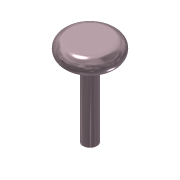
# Autodesk Inventor part: screw
Saved by Autodesk Inventor 2022 Beta2 (Build 260130000, 130) ContinuousBuild 0
## iProperties
Shininess: 64.0
Length Units: 11272
Angle Units: 11279
Time Units: 11290
Mass Units: 11286
Length Display Precision: 3
Angle Display Precision: 2
Created: 2002-02-11
Part Number: screw
Document SubType Name: Modeling
Designer: Administrator
Density: 1 g/cm^3
Material: Generic
Appearance: Pink Champagne
Density: 0.0
Volumn: 0.0
Area: 0.0
PropertySet Name: Model Information
Control State: 0
Master: False
Checked Out: False
Author: Administrator
Autodesk Inventor part; units mm, degrees
ref_plane "YZ Plane" through (0, 0, 0) normal (1, 0, 0) x (0, 1, 0)
ref_plane "XZ Plane" through (0, 0, 0) normal (0, 1, 0) x (-1, 0, 0)
ref_plane "XY Plane" through (0, 0, 0) normal (0, 0, 1) x (1, 0, 0)
sketch "Sketch1" plane through (0, 0, 0) normal (0, 0, 1) x (1, 0, 0)
  line L0 (-5.9224, 6.0856) -> (-5.9224, -9.7894)
  line L1 (-5.9224, -9.7894) -> (-4.6778, -9.7894)
  line L2 (-4.6778, -9.7894) -> (-4.6778, 2.9106)
  line L3 (-4.6778, 2.9106) -> (-2.7474, 2.9106)
  arc A0 (-2.7474, 2.9106) -> (-2.7474, 6.0856) centre (-2.7474, 4.4981) ccw
  line L4 (-2.7474, 6.0856) -> (-5.9224, 6.0856)
  dimension "d0" = 12.7
  dimension "d1" = 1.5875
  dimension "d2" = 1.2446
  dimension "d3" = 3.175
  constraints: 10 end point, 3 parallel, 2 point on circle, 2 tangent, 1 centre point, 1 perpendicular, 1 vertical
  measures "d0" distance of L1.end L2.end
  measures "d1" radius of A0
  measures "d2" distance of L0.end L1.end
  measures "d3" distance of L4.start L0.start
revolve "Revolution1" add sketch "Sketch1" angle 360 about axis through (-5.9224, 6.0856, 0) along (0, -1, 0)
body "Solid1"
